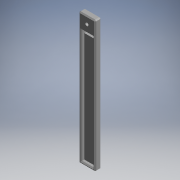
# Autodesk Inventor part: 風力
Saved by Autodesk Inventor 2021 (Build 250183000, 183)
## iProperties
Part Number: 風力
Material: 一般
Document SubType Name: 塑型
Designer: aura0
Appearance: 預設
Author: aura0
Autodesk Inventor part; units mm, degrees
ref_plane "YZ 平面" through (0, 0, 0) normal (1, 0, 0) x (0, 1, 0)
ref_plane "XZ 平面" through (0, 0, 0) normal (0, 1, 0) x (-1, 0, 0)
ref_plane "XY 平面" through (0, 0, 0) normal (0, 0, 1) x (1, 0, 0)
sketch "草圖1" plane through (0, 0, 0) normal (0, 0, 1) x (1, 0, 0)
  line L0 (-8, -63.5) -> (8, -63.5)
  line L1 (8, -63.5) -> (8, 63.5)
  line L2 (8, 63.5) -> (-8, 63.5)
  line L3 (-8, 63.5) -> (-8, -63.5)
  line L4 (-8, -63.5) -> (8, 63.5) construction
  line L5 (8, -63.5) -> (-8, 63.5) construction
  point P0 (0, 0)
  dimension "d0" = 16
  dimension "d1" = 127
  constraints: 12 end point, 2 midpoint, 2 parallel, 1 horizontal, 1 perpendicular
  measures "d0" distance of L2.end L1.end
  measures "d1" distance of L1.end L0.end
extrude "擠出1" add sketch "草圖1" along normal blind 6
sketch "草圖2" plane through (0, 0, 6) normal (0, 0, 1) x (1, 0, 0)
  line L0 (-5.5, -61) -> (5.5, -61)
  line L1 (5.5, -61) -> (5.5, 49)
  line L2 (5.5, 49) -> (-5.5, 49)
  line L3 (-5.5, 49) -> (-5.5, -61)
  line L4 (-5.5, -61) -> (5.5, 49) construction
  line L5 (5.5, -61) -> (-5.5, 49) construction
  line L6 (-8, -63.5) -> (8, -63.5) projected
  line L7 (8, -63.5) -> (8, 63.5) projected
  point P0 (0, 0)
  point P1 (0, -6)
  dimension "d4" = 11
  dimension "d5" = 110
  dimension "d6" = 2.5
  dimension "d7" = 2.5
  constraints: 12 end point, 2 midpoint, 2 parallel, 1 horizontal, 1 perpendicular
  measures "d4" distance of L2.end L1.end
  measures "d5" distance of L1.end L0.end
  measures "d6" distance between parallel lines of L0 L6
  measures "d7" distance between parallel lines of L7 L1
extrude "擠出2" cut sketch "草圖2" against normal blind 3
sketch "草圖3" plane through (0, 0, 3) normal (0, 0, 1) x (1, 0, 0)
  line L0 (-5.5, 49) -> (5.5, 49)
  line L1 (5.5, 49) -> (5.5, 45)
  line L2 (5.5, 45) -> (-5.5, 45)
  line L3 (-5.5, 45) -> (-5.5, 49)
  line L4 (-5.5, 49) -> (5.5, 45) construction
  line L5 (5.5, 49) -> (-5.5, 45) construction
  line L6 (-5.5, 49) -> (5.5, 49) projected
  line L7 (-5.5, -61) -> (-5.5, 49) projected
  point P0 (0, 0)
  point P1 (0, 47)
  dimension "d10" = 11
  dimension "d11" = 4
  dimension "d12" = 0
  dimension "d13" = 0
  constraints: 12 end point, 2 midpoint, 2 parallel, 1 horizontal, 1 perpendicular
  measures "d10" distance of L1.end L2.end
  measures "d11" distance of L0.end L1.end
  measures "d12" distance between parallel lines of L6 L0
  measures "d13" distance between parallel lines of L7 L3
extrude "擠出3" cut sketch "草圖3" against normal blind 3
sketch "草圖4" plane through (0, 0, 6) normal (0, 0, 1) x (1, 0, 0)
  circle A0 centre (0, 56.5) radius 1.5
  line L0 (8, 63.5) -> (-8, 63.5) projected
  line L1 (-8, 63.5) -> (-8, -63.5) projected
  point P0 (0, 0)
  dimension "d16" = 7
  dimension "d17" = 8
  dimension "d18" = 3
  constraints: 1 centre point
  measures "d16" distance from line of L0 A0.centre
  measures "d17" distance from line of L1 A0.centre
  measures "d18" diameter of A0
extrude "擠出4" cut sketch "草圖4" against normal blind 6
chamfer "倒角1" distance 1 angle 45 16 edges at (-5.5, -6, 6) (-8, 0, 6) (8, 0, 6) (5.5, -6, 6) (0, 49, 6) (0, -61, 6) (0, -63.5, 6) (0, 63.5, 6) (8, 63.5, 3) (-8, 63.5, 3) (8, -63.5, 3) (-8, -63.5, 3) (-8, 0, 0) (0, -63.5, 0) (8, 0, 0) (0, 63.5, 0)
sketch "草圖5" plane through (0, 0, 0) normal (0, 0, -1) x (-1, 0, 0)
  circle A0 centre (0, 56.5) radius 3
  line L0 (7, 63.5) -> (-7, 63.5) projected
  line L1 (8, -62.5) -> (8, 62.5) projected
  point P0 (0, 0)
  dimension "d24" = 6
  dimension "d25" = 7
  dimension "d26" = 8
  constraints: 1 centre point
  measures "d24" diameter of A0
  measures "d25" distance from line of L0 A0.centre
  measures "d26" distance from line of L1 A0.centre
extrude "擠出5" cut sketch "草圖5" against normal blind 2
chamfer "倒角2" distance 1 angle 45 2 edges at (0, 45, 0) (0, 49, 0)
chamfer "倒角3" distance 1 angle 45 1 edges at (-5.5, 44.5, 0)
chamfer "倒角4" distance 1 angle 45 1 edges at (5.5, 44.5, 0)
